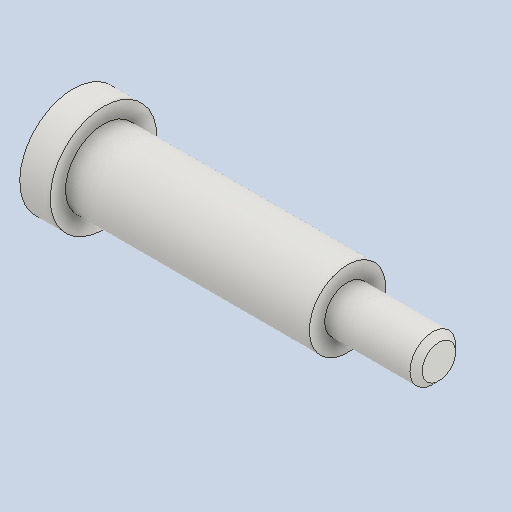
# Autodesk Inventor part: Вал
Saved by Autodesk Inventor 2022 (Build 260153000, 153)
## iProperties
CustomPartVersion: 1
Created: 2021-10-26
Part Number: Вал
Material: Steel
Document SubType Name: Modeling
Designer: RaNSiD
Density: 1 g/cm^3
Appearance: Steel
Length: 120,000 мм
Author: RaNSiD
Autodesk Inventor part; units mm, degrees
ref_plane "Начальная плоскость" through (0, 0, 0) normal (1, 0, 0) x (0, 1, 0)
ref_plane "XZ Plane" through (0, 0, 0) normal (0, 1, 0) x (-1, 0, 0)
ref_plane "XY Plane" through (0, 0, 0) normal (0, 0, 1) x (1, 0, 0)
sketch "Основной эскиз" plane through (0, 0, 0) normal (0, 0, 1) x (1, 0, 0)
  line L0 (0, 0) -> (120, 0)
  line L1 (0, 0) -> (0, 17.5)
  line L2 (10, 17.5) -> (10, 12.5)
  line L3 (0, 17.5) -> (10, 17.5)
  line L4 (90, 12.5) -> (90, 7.5)
  line L5 (10, 12.5) -> (90, 12.5)
  line L6 (120, 7.5) -> (120, 0)
  line L7 (90, 7.5) -> (120, 7.5)
  dimension "d3" = 35
  dimension "d4" = 25
  dimension "d5" = 15
  constraints: 16 end point, 4 vertical, 2 horizontal
  measures "d3" diameter of L3 L0
  measures "d4" diameter of L5 L0
  measures "d5" diameter of L7 L0
revolve "Вращение1" add sketch "Основной эскиз" angle 360 about axis through (0, 0, 0) along (1, 0, 0)
chamfer "Фаска1" distance 2 angle 45 1 edges at (120, -7.5, 0) measured on face at (100, 7.4757, -0.6035)
